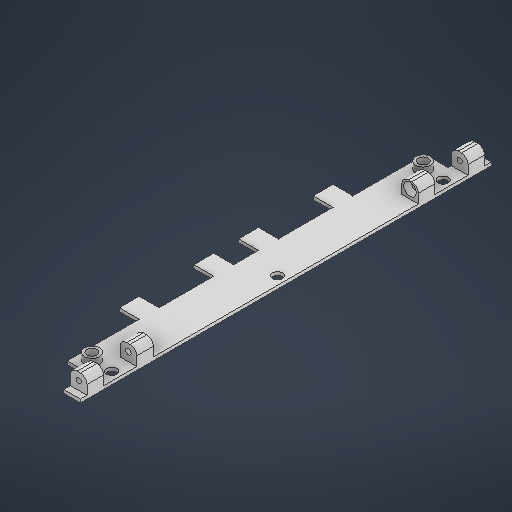
# Autodesk Inventor part: zawiasv2
Saved by Autodesk Inventor 2026.2 (Build 302298010, 298A)
## iProperties
Created: 2026-05-22
Part Number: zawiasv2
Material: Ogólny
Document SubType Name: Modeling
Designer: karol
Density: 1 g/cm^3
Appearance: Domyślna
Author: karol
Autodesk Inventor part; units mm, degrees
ref_plane "YZ Plane" through (0, 0, 0) normal (1, 0, 0) x (0, 1, 0)
ref_plane "XZ Plane" through (0, 0, 0) normal (0, 1, 0) x (-1, 0, 0)
ref_plane "XY Plane" through (0, 0, 0) normal (0, 0, 1) x (1, 0, 0)
sketch "Szkic1" plane through (0, 0, 0) normal (0, 1, 0) x (-1, 0, 0)
  line L0 (0, 0) -> (5, 0)
  line L1 (5, 0) -> (5, -62)
  line L2 (5, -62) -> (0, -62)
  line L3 (0, -62) -> (0, 0)
  line L4 (0, 0) -> (5, 0)
  line L5 (5, 0) -> (5, 62)
  line L6 (5, 62) -> (0, 62)
  line L7 (0, 62) -> (0, 0)
  line L8 (0, 62) -> (5, 62)
  line L9 (5, 62) -> (5, 60)
  line L10 (5, 60) -> (0, 60)
  line L11 (0, 60) -> (0, 62)
  line L12 (5, 60) -> (0, 60)
  line L13 (0, 60) -> (0, 55)
  line L14 (0, 55) -> (5, 55)
  line L15 (5, 55) -> (5, 60)
  line L16 (5, 55) -> (0, 55)
  line L17 (0, 55) -> (0, 45)
  line L18 (0, 45) -> (5, 45)
  line L19 (5, 45) -> (5, 55)
  line L20 (5, 45) -> (0, 45)
  line L21 (0, 45) -> (0, 40)
  line L22 (0, 40) -> (5, 40)
  line L23 (5, 40) -> (5, 45)
  line L24 (0, 40) -> (5, 40)
  line L25 (5, 40) -> (5, 38)
  line L26 (5, 38) -> (0, 38)
  line L27 (0, 38) -> (0, 40)
  line L28 (0, -62) -> (5, -62)
  line L29 (5, -62) -> (5, -60)
  line L30 (5, -60) -> (0, -60)
  line L31 (0, -60) -> (0, -62)
  line L32 (0, -60) -> (5, -60)
  line L33 (5, -60) -> (5, -55)
  line L34 (5, -55) -> (0, -55)
  line L35 (0, -55) -> (0, -60)
  line L36 (0, -55) -> (5, -55)
  line L37 (5, -55) -> (5, -45)
  line L38 (5, -45) -> (0, -45)
  line L39 (0, -45) -> (0, -55)
  line L40 (0, -45) -> (5, -45)
  line L41 (5, -45) -> (5, -40)
  line L42 (5, -40) -> (0, -40)
  line L43 (0, -40) -> (0, -45)
  line L44 (0, -40) -> (5, -40)
  line L45 (5, -40) -> (5, -38)
  line L46 (5, -38) -> (0, -38)
  line L47 (0, -38) -> (0, -40)
  point P0 (0, -45)
  point P1 (0, -55)
  point P2 (5, 40)
  point P3 (5, 55)
  point P4 (0, 60)
  dimension "d0" = 5
  dimension "d1" = 62
  dimension "d2" = 62
  dimension "d3" = 2
  dimension "d4" = 5
  dimension "d5" = 10
  dimension "d6" = 5
  dimension "d7" = 2
  dimension "d8" = 2
  dimension "d9" = 5
  dimension "d10" = 10
  dimension "d11" = 5
  dimension "d12" = 2
  constraints: 96 end point, 24 parallel, 12 horizontal, 12 perpendicular, 11 point on line
  measures "d0" distance of L1.end L2.end
  measures "d1" distance of L0.end L1.end
  measures "d2" distance of L5.end L4.end
  measures "d3" distance of L8.end L9.end
  measures "d4" distance of L13.end L12.end
  measures "d5" distance of L17.end L16.end
  measures "d6" distance of L21.end L20.end
  measures "d7" distance of L24.end L25.end
  measures "d8" distance of L29.end L28.end
  measures "d9" distance of L33.end L32.end
  measures "d10" distance of L37.end L36.end
  measures "d11" distance of L41.end L40.end
  measures "d12" distance of L45.end L44.end
extrude "Wyciągnięcie proste1" add sketch "Szkic1" against normal blind 0.8
extrude "Wyciągnięcie proste2" add sketch "Szkic1" along normal blind 5 contours L42 L1 L38 L3 | L7 L18 L5 L22 | L34 L1 L30 L3 | L7 L10 L5 L14
sketch "Szkic2" plane through (0, 0, 40) normal (0, 0, -1) x (-1, 0, 0)
  circle A0 centre (2.5, 2.8) radius 1.9
  circle A1 centre (2.5, 2.8) radius 0.8
  line L0 (5, 0) -> (5, 5) projected
  line L1 (0, 5) -> (5, 5) projected
  point P0 (0, 0)
  point P1 (5, 2.5)
  dimension "d17" = 3.8
  dimension "d18" = 1.6
  dimension "d19" = 2.5
  dimension "d20" = 2.2
  constraints: 2 centre point, 1 coincident, 1 midpoint
  measures "d17" diameter of A0
  measures "d18" diameter of A1
  measures "d19" horizontal distance of point (5, 2.5) A0.centre
  measures "d20" distance from line of L1 A0.centre
extrude "Wyciągnięcie proste3" cut sketch "Szkic2" against normal blind 2.2 contours A0 | A1
extrude "Wyciągnięcie proste4" cut sketch "Szkic2" against normal blind 20 contours A1
thread "Gwint1" size "M2x0.4" class "6H" standard "ANSI Metric M Profile" full length
sketch "Szkic3" plane through (-5, 0, -40) normal (0, 0, 1) x (1, 0, 0)
  circle A0 centre (2.5, 2.8) radius 0.8 projected
  circle A1 centre (2.5, 2.8) radius 1.9
  circle A2 centre (2.5, 2.8) radius 0.8
  point P0 (5, 0)
  dimension "d27" = 3.8
  dimension "d28" = 1.6
  constraints: 2 centre point, 2 coincident
  measures "d27" diameter of A1
  measures "d28" diameter of A2
extrude "Wyciągnięcie proste5" cut sketch "Szkic3" against normal blind 2.2 contours A0 | A1
extrude "Wyciągnięcie proste6" cut sketch "Szkic3" against normal blind 20 contours A0
thread "Gwint2" size "M2x0.4" class "6H" standard "ANSI Metric M Profile" full length
fillet "Zaokrąglenie1" radius 2 8 edges at (-5, 5, 57.5) (0, 5, 57.5) (0, 5, 42.5) (-5, 5, 42.5) (0, 5, -42.5) (-5, 5, -42.5) (0, 5, -57.5) (-5, 5, -57.5)
sketch "Szkic4" plane through (0, 0, 0) normal (0, 1, 0) x (1, 0, 0)
  circle A0 centre (-2.5, -50) radius 1.55
  circle A1 centre (-2.5, 50) radius 1.55
  circle A2 centre (-2.5, 0) radius 1.55
  line L0 (-5, -45) -> (-5, -55) projected
  line L1 (-3, -45) -> (-2, -45) projected
  line L2 (-2, 45) -> (-3, 45) projected
  line L3 (-5, 55) -> (-5, 45) projected
  line L4 (-5, 40) -> (-5, -40) projected
  line L5 (0, 62) -> (-5, 62) projected
  point P0 (0, 0)
  point P1 (-2.5, -45)
  point P2 (-2.5, 45)
  point P3 (-5, 50)
  point P4 (-2.5, 62)
  dimension "d36" = 3.1
  dimension "d37" = 2.5
  dimension "d38" = 5
  dimension "d39" = 5
  dimension "d40" = 2.5
  dimension "d41" = 3.1
  dimension "d42" = 2.5
  dimension "d43" = 62
  dimension "d44" = 3.1
  constraints: 4 midpoint, 3 centre point
  measures "d36" diameter of A0
  measures "d37" distance from line of L0 A0.centre
  measures "d38" distance of point (-2.5, -45) A0.centre
  measures "d39" distance of point (-2.5, 45) A1.centre
  measures "d40" distance of point (-5, 50) A1.centre
  measures "d41" diameter of A1
  measures "d42" distance from line of L4 A2.centre
  measures "d43" distance of point (-2.5, 62) A2.centre
  measures "d44" diameter of A2
extrude "Wyciągnięcie proste7" cut sketch "Szkic4" against normal blind 0.8
sketch "Sketch7" plane through (-5, -0.8, -62) normal (-1, 0, 0) x (0, 0, 1)
  line L0 (0, 0) -> (124, 0)
  line L1 (124, 0) -> (124, 0.8)
  line L2 (124, 0.8) -> (0, 0.8)
  line L3 (0, 0.8) -> (0, 0)
  point P0 (62, 0.8)
  constraints: 8 end point, 2 parallel, 1 horizontal, 1 perpendicular
extrude "Extrusion10" add sketch "Sketch7" along normal blind 7
sketch "Sketch8" plane through (0, -0.8, 62) normal (0, 0, 1) x (1, 0, 0)
  line L0 (-12, 0.8) -> (0, 0.8) projected
  line L1 (0, 0) -> (-12, 0) projected
  line L2 (-12, 0.8) -> (-5, 0.8)
  line L3 (-5, 0.8) -> (-5, 0)
  line L4 (-5, 0) -> (-12, 0)
  line L5 (-12, 0) -> (-12, 0.8)
  dimension "d59" = 7
  constraints: 8 end point, 2 parallel, 1 horizontal, 1 perpendicular, 1 point on line
  measures "d59" distance of L3.end L4.end
extrude "Extrusion11" cut sketch "Sketch8" against normal blind 8
sketch "Sketch9" plane through (0, -0.8, -62) normal (0, 0, -1) x (-1, 0, 0)
  line L0 (5, 0.8) -> (5, 0) projected
  line L1 (0, 0.8) -> (12, 0.8) projected
  line L2 (0, 0.8) -> (0, 0) projected
  line L3 (0, 0) -> (12, 0) projected
  line L4 (12, 0.8) -> (12, 0) projected
  line L5 (5, 0.8) -> (12, 0.8)
  line L6 (12, 0.8) -> (12, 0)
  line L7 (12, 0) -> (5, 0)
  line L8 (5, 0) -> (5, 0.8)
  point P0 (0, 0.8)
  constraints: 8 end point, 2 parallel, 1 horizontal, 1 perpendicular
extrude "Extrusion12" cut sketch "Sketch9" against normal blind 8 contours L1 L4 L3 L0
sketch "Sketch10" plane through (0, 0, 0) normal (0, 1, 0) x (1, 0, 0)
  line L0 (-12, -54) -> (-12, 54) projected
  line L1 (-12, 32.25) -> (-18, 32.25)
  line L2 (-18, 32.25) -> (-18, 26.25)
  line L3 (-18, 26.25) -> (-12, 26.25)
  line L4 (-12, 26.25) -> (-12, 32.25)
  line L5 (-12, -32.25) -> (-18, -32.25)
  line L6 (-18, -32.25) -> (-18, -26.25)
  line L7 (-18, -26.25) -> (-12, -26.25)
  line L8 (-12, -26.25) -> (-12, -32.25)
  line L9 (-12, -54) -> (-5, -54) projected
  point P0 (0, 0)
  point P1 (-15, 32.25)
  point P2 (-12, 26.25)
  dimension "d64" = 6
  dimension "d65" = 6
  dimension "d66" = 6
  dimension "d67" = 6
  dimension "d68" = 21.75
  dimension "d69" = 21.75
  constraints: 16 end point, 4 parallel, 2 horizontal, 2 perpendicular, 2 point on line, 1 midpoint
  measures "d64" distance of L3.end L2.end
  measures "d65" distance of L1.end L2.end
  measures "d66" distance of L6.end L7.end
  measures "d67" distance of L5.end L6.end
  measures "d68" vertical distance of L0.end point (-15, 32.25)
  measures "d69" distance between parallel lines of L5 L9
extrude "Extrusion13" add sketch "Sketch10" against normal blind 0.8
sketch "Sketch11" plane through (0, 0, 0) normal (0, 1, 0) x (1, 0, 0)
  line L0 (-5, 62) -> (-5, 60) projected
  line L1 (-5, 60) -> (0, 60) projected
  line L2 (0, 60) -> (0, 62) projected
  line L3 (0, 62) -> (-5, 62) projected
  line L4 (-5, 55) -> (-5, 54) projected
  line L5 (-5, 54) -> (-12, 54) projected
  line L6 (-12, 32.25) -> (-12, 54) projected
  line L7 (-12, 32.25) -> (-18, 32.25) projected
  line L8 (-18, 32.25) -> (-18, 26.25) projected
  line L9 (-18, 26.25) -> (-12, 26.25) projected
  line L10 (-12, -26.25) -> (-12, 26.25) projected
  line L11 (-12, -26.25) -> (-18, -26.25) projected
  line L12 (-18, -26.25) -> (-18, -32.25) projected
  line L13 (-18, -32.25) -> (-12, -32.25) projected
  line L14 (-12, -54) -> (-12, -32.25) projected
  line L15 (-12, -54) -> (-5, -54) projected
  line L16 (-5, -54) -> (-5, -55) projected
  line L17 (-5, -55) -> (0, -55) projected
  line L18 (0, -55) -> (0, -45) projected
  line L19 (0, -45) -> (-5, -45) projected
  line L20 (-5, -40) -> (-5, -45) projected
  line L21 (-5, -40) -> (0, -40) projected
  line L22 (0, -40) -> (0, 40) projected
  line L23 (0, 40) -> (-5, 40) projected
  line L24 (-5, 45) -> (-5, 40) projected
  line L25 (-5, 45) -> (0, 45) projected
  line L26 (0, 45) -> (0, 55) projected
  line L27 (0, 55) -> (-5, 55) projected
  circle A0 centre (-2.5, -50) radius 1.55 projected
  circle A1 centre (-2.5, 50) radius 1.55 projected
  circle A2 centre (-2.5, 0) radius 1.55 projected
  line L28 (-5, 62) -> (-5, 60) projected
  line L29 (-5, 60) -> (0, 60) projected
  line L30 (0, 60) -> (0, 62) projected
  line L31 (0, 62) -> (-5, 62) projected
  line L32 (-5, 55) -> (-5, 54) projected
  line L33 (-5, 54) -> (-12, 54) projected
  line L34 (-12, 32.25) -> (-12, 54) projected
  line L35 (-12, 32.25) -> (-18, 32.25) projected
  line L36 (-18, 32.25) -> (-18, 26.25) projected
  line L37 (-18, 26.25) -> (-12, 26.25) projected
  line L38 (-12, -26.25) -> (-12, 26.25) projected
  line L39 (-12, -26.25) -> (-18, -26.25) projected
  line L40 (-18, -26.25) -> (-18, -32.25) projected
  line L41 (-18, -32.25) -> (-12, -32.25) projected
  line L42 (-12, -54) -> (-12, -32.25) projected
  line L43 (-12, -54) -> (-5, -54) projected
  line L44 (-5, -54) -> (-5, -55) projected
  line L45 (-5, -55) -> (0, -55) projected
  line L46 (0, -55) -> (0, -45) projected
  line L47 (0, -45) -> (-5, -45) projected
  line L48 (-5, -40) -> (-5, -45) projected
  line L49 (-5, -40) -> (0, -40) projected
  line L50 (0, -40) -> (0, 40) projected
  line L51 (0, 40) -> (-5, 40) projected
  line L52 (-5, 45) -> (-5, 40) projected
  line L53 (-5, 45) -> (0, 45) projected
  line L54 (0, 45) -> (0, 55) projected
  line L55 (0, 55) -> (-5, 55) projected
  circle A3 centre (-2.5, -50) radius 1.55 projected
  circle A4 centre (-2.5, 50) radius 1.55 projected
  circle A5 centre (-2.5, 0) radius 1.55 projected
  line L56 (-5, -60) -> (-5, -62) projected
  line L57 (-5, -62) -> (0, -62) projected
  line L58 (0, -62) -> (0, -60) projected
  line L59 (0, -60) -> (-5, -60) projected
  point P0 (0, 0)
extrude "Extrusion14" add sketch "Sketch11" along normal blind 0.2
sketch "Sketch12" plane through (0, 0.2, 0) normal (0, 1, 0) x (1, 0, 0)
  line L0 (-12, 26.25) -> (-12, -26.25) projected
  line L1 (-12, 9.75) -> (-18, 9.75)
  line L2 (-18, 9.75) -> (-18, 3.75)
  line L3 (-18, 3.75) -> (-12, 3.75)
  line L4 (-12, 3.75) -> (-12, 9.75)
  line L5 (-12, -9.75) -> (-18, -9.75)
  line L6 (-18, -9.75) -> (-18, -3.75)
  line L7 (-18, -3.75) -> (-12, -3.75)
  line L8 (-12, -3.75) -> (-12, -9.75)
  line L9 (-18, 26.25) -> (-12, 26.25) projected
  line L10 (-12, -26.25) -> (-18, -26.25) projected
  point P0 (0, 0)
  point P1 (-15, 9.75)
  point P2 (-15, 26.25)
  point P3 (-15, -26.25)
  point P4 (-15, -9.75)
  point P5 (-12, -3.75)
  point P6 (-12, 3.75)
  dimension "d76" = 6
  dimension "d77" = 6
  dimension "d78" = 6
  dimension "d79" = 6
  dimension "d84" = 16.5
  dimension "d85" = 16.5
  constraints: 16 end point, 4 midpoint, 4 parallel, 2 horizontal, 2 perpendicular, 2 point on line
  measures "d76" distance of L3.end L2.end
  measures "d77" distance of L2.end L1.end
  measures "d78" distance of L6.end L7.end
  measures "d79" distance of L5.end L6.end
  measures "d84" distance between parallel lines of L10 L5
  measures "d85" distance between parallel lines of L9 L1
extrude "Extrusion15" add sketch "Sketch12" against normal blind 1
sketch "Sketch13" plane through (0, 0.2, 0) normal (0, 1, 0) x (1, 0, 0)
  circle A0 centre (-8.5, -50) radius 1.5
  line L0 (-12, -54) -> (-5, -54) projected
  line L1 (-12, -32.25) -> (-12, -54) projected
  circle A1 centre (-8.5, 50) radius 1.5
  line L2 (-5, 54) -> (-12, 54) projected
  line L3 (-12, 54) -> (-12, 32.25) projected
  circle A2 centre (-8.5, -50) radius 2.3
  circle A3 centre (-8.5, 50) radius 2.3
  point P0 (0, 0)
  dimension "d86" = 3
  dimension "d87" = 4
  dimension "d88" = 3.5
  dimension "d89" = 3
  dimension "d90" = 4
  dimension "d91" = 3.5
  dimension "d92" = 4.6
  dimension "d93" = 4.6
  constraints: 4 centre point, 2 coincident
  measures "d86" diameter of A0
  measures "d87" distance from line of L0 A0.centre
  measures "d88" distance from line of L1 A0.centre
  measures "d89" diameter of A1
  measures "d90" distance from line of L2 A1.centre
  measures "d91" distance from line of L3 A1.centre
  measures "d92" diameter of A2
  measures "d93" diameter of A3
extrude "Extrusion16" add sketch "Sketch13" along normal blind 2
extrude "Extrusion17" cut sketch "Sketch13" against normal blind 0.2 contours A0 | A1
